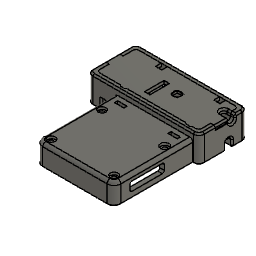
Arduino Portenta H7 and OLED Case For ML Car v32 (Autodesk Fusion 360 design; units mm, degrees)
Autodesk Fusion 360 part; units mm, degrees
note: some values were not read from the file. Chosen so that the rebuilt part matches the saved one: which face or edge a step refers to; which pieces of a blend or face edit are solid. Set by a fixed rule: which sketch regions a step uses; the direction of a hole.
(part 1 of 2)
sketch "Sketch1" plane through (0, 0, 0) normal (0, 0, 1) x (1, 0, 0)
  line L0 (1.5, 0) -> (43, 0)
  line L1 (44.5, 1.5) -> (44.5, 35.5)
  line L2 (43, 37) -> (1.5, 37)
  line L3 (0, 35.5) -> (0, 1.5)
  circle A0 centre (2, 34.875) radius 1.5
  circle A1 centre (42.5, 34.875) radius 1.5
  circle A2 centre (42.5, 2.125) radius 1.5
  circle A3 centre (2, 2.125) radius 1.5
  arc A4 (1.5, 37) -> (0, 35.5) centre (1.5, 35.5) ccw
  arc A5 (44.5, 35.5) -> (43, 37) centre (43, 35.5) ccw
  arc A6 (0, 1.5) -> (1.5, 0) centre (1.5, 1.5) ccw
  arc A7 (43, 0) -> (44.5, 1.5) centre (43, 1.5) ccw
  line L4 (1.5, -3) -> (43, -3)
  arc A8 (43, -3) -> (47.5, 1.5) centre (43, 1.5) ccw
  line L5 (47.5, 1.5) -> (47.5, 40)
  line L6 (47.5, 40) -> (-3, 40)
  line L7 (-3, 40) -> (-3, 1.5)
  arc A9 (-3, 1.5) -> (1.5, -3) centre (1.5, 1.5) ccw
  circle A10 centre (42.5, 2.125) radius 2.5
  circle A11 centre (2, 2.125) radius 2.5
  circle A12 centre (42.5, 34.875) radius 2.5
  circle A13 centre (2, 34.875) radius 2.75
  point P0 (44.5, 0)
  point P1 (0, 37)
  dimension "d1" = 44.5
  dimension "d2" = 37
  dimension "d3" = 3
  dimension "d4" = 2
  dimension "d5" = 2.125
  dimension "d6" = 2
  dimension "d7" = 2.125
  dimension "d9" = 1.5
  dimension "d16" = 1
  dimension "d17" = 1
  dimension "d19" = 1
  dimension "d372" = 5.5
  constraint horizontal L0
  constraint vertical L1
  constraint horizontal L2
  constraint vertical L3
  constraint equal A1 A3
  constraint equal A1 A2
  constraint equal A0 A2
  constraint horizontal A0.centre A1.centre
  constraint vertical A0.centre A3.centre
  constraint horizontal A2.centre A3.centre
  constraint vertical A1.centre A2.centre
  constraint coincident P1 L2
  constraint coincident P1 L3
  constraint tangent L2 A4
  constraint tangent L3 A4
  constraint tangent L1 A5
  constraint tangent L2 A5
  constraint equal A4 A5
  constraint coincident origin L0
  constraint coincident origin L3
  constraint tangent L0 A6
  constraint tangent L3 A6
  constraint equal A4 A6
  constraint coincident P0 L0
  constraint coincident P0 L1
  constraint tangent L0 A7
  constraint tangent L1 A7
  constraint equal A4 A7
  constraint parallel L0 L4
  constraint concentric A7 A8
  constraint parallel L1 L5
  constraint parallel L2 L6
  constraint parallel L3 L7
  constraint concentric A6 A9
  constraint tangent L4 A9
  constraint tangent L4 A8
  constraint tangent A8 L5
  constraint tangent L7 A9
  constraint concentric A0 A13
  measures "d1" distance of origin P0
  measures "d2" distance of origin P1
  measures "d3" diameter of A0
  measures "d4" distance of L3 A0.centre
  measures "d5" distance of L2 A0.centre
  measures "d6" distance of L1 A1.centre
  measures "d7" distance of L0 A3.centre
  measures "d9" radius of A4
  measures "d372" diameter of A13
extrude "Extrude1" add sketch "Sketch1" along normal blind 14 contours L0 L3 A6 A11 | L0 L3 A6 A11 | L0 L1 L2 L3 A10 A11 A12 A13 | L0 L1 A7 A10 | L0 L1 A7 A10 | L2 L3 A4 A13 | L2 L3 A4 A13 | L1 L2 A5 A12 | L1 L2 A5 A12 | A0 | A1 | A2 | A3 | L4 A8 L5 L6 L7 A9 makes body 1
extrude "Extrude2" cut sketch "Sketch1" along normal up to surface (10 mm away) from surface at 4 contours L0 L3 A6 A11 | L0 L1 L2 L3 A10 A11 A12 A13 | L0 L1 A7 A10 | L2 L3 A4 A13 | L1 L2 A5 A12 | A0 | A1 | A2 | A3 picked at (2.3836, 0.2209) picked at (42.1164, 0.2209) picked at (2.5264, 36.7791) picked at (42.1164, 36.7791) bodies 1
extrude "Extrude3" cut sketch "Sketch1" along normal through all contours A0 | A1 | A2 | A3 bodies 1
extrude "Extrude28" cut sketch "Sketch1" along normal blind 1.55 contours L0 L3 A6 A11 | L0 L3 A6 A11 | L0 L1 A7 A10 | L0 L1 A7 A10 | L2 L3 A4 A13 | L2 L3 A4 A13 | L1 L2 A5 A12 | L1 L2 A5 A12 bodies 1
extrude "Extrude5" add 1 faces at (30.6667, 40, 4.6667) along direction (0, 1, 0) blind 8 on bodies 1 bodies 1
sketch "Sketch3" plane through (44.5, 0, 0) normal (-1, 0, 0) x (0, -1, 0)
  line L0 (-35.5, 4) -> (-1.5, 4)
  line L1 (-1.5, 4) -> (-1.5, 14)
  line L2 (-1.5, 14) -> (-35.5, 14)
  line L3 (-35.5, 14) -> (-35.5, 4)
  line L4 (-30.75, 4) -> (-30.75, 8)
  line L5 (-29.75, 9) -> (-7.25, 9)
  line L6 (-6.25, 8) -> (-6.25, 4)
  line L7 (-6.25, 4) -> (-30.75, 4)
  arc A0 (-29.75, 9) -> (-30.75, 8) centre (-29.75, 8) ccw
  arc A1 (-6.25, 8) -> (-7.25, 9) centre (-7.25, 8) ccw
  dimension "d30" = 4.75
  dimension "d31" = 4.75
  dimension "d33" = 5
  dimension "d35" = 1
  constraint horizontal L5
  constraint vertical L6
  constraint horizontal L7
  constraint vertical L4
  constraint tangent L4 A0
  constraint tangent L5 A0
  constraint tangent L5 A1
  constraint tangent L6 A1
  constraint equal A0 A1
  constraint collinear L0 L7
  measures "d30" distance of L3 L4
  measures "d31" distance of L1 L6
  measures "d33" distance of L5 L7
  measures "d35" radius of A0
sketch "Sketch18" plane through (0, 0, 0) normal (1, 0, 0) x (0, 1, 0)
  line L0 (1.5, 4) -> (35.5, 4)
  line L1 (35.5, 4) -> (35.5, 14)
  line L2 (35.5, 14) -> (1.5, 14)
  line L3 (1.5, 14) -> (1.5, 4)
  line L4 (8.625, 4) -> (28.375, 4)
  line L5 (29.625, 5.25) -> (29.625, 8.5)
  line L6 (28.375, 9.75) -> (8.625, 9.75)
  line L7 (7.375, 8.5) -> (7.375, 5.25)
  arc A0 (8.625, 9.75) -> (7.375, 8.5) centre (8.625, 8.5) ccw
  arc A1 (29.625, 8.5) -> (28.375, 9.75) centre (28.375, 8.5) ccw
  arc A2 (28.375, 4) -> (29.625, 5.25) centre (28.375, 5.25) ccw
  arc A3 (7.375, 5.25) -> (8.625, 4) centre (8.625, 5.25) ccw
  point P0 (7.375, 4)
  point P1 (7.375, 9.75)
  point P2 (2.125, 0)
  point P3 (34.875, 0)
  dimension "d203" = 5.75
  dimension "d204" = 5.25
  dimension "d205" = 5.25
  dimension "d206" = 1.25
  constraint horizontal L4
  constraint vertical L5
  constraint horizontal L6
  constraint vertical L7
  constraint coincident L0 P0
  constraint coincident P1 L6
  constraint coincident P1 L7
  constraint tangent L6 A0
  constraint tangent L7 A0
  constraint tangent L6 A1
  constraint tangent L5 A1
  constraint equal A0 A1
  constraint tangent L4 A2
  constraint tangent L5 A2
  constraint equal A0 A2
  constraint coincident P0 L4
  constraint coincident P0 L7
  constraint tangent L4 A3
  constraint tangent L7 A3
  constraint equal A0 A3
  measures "d203" distance of P0 P1
  measures "d204" distance of L5 P3
  measures "d205" distance of L7 P2
  measures "d206" radius of A0
extrude "Extrude6" cut sketch "Sketch18" against normal through all contours L0 L4 L5 L6 L7 A0 A1 A2 A3 bodies 1
extrude "Extrude7" cut sketch "Sketch3" against normal through all contours L0 L4 L5 L6 L7 A0 A1 bodies 1
fillet "Fillet1" radius 2 5 edges at (-3, 24.75, 0) (-1.682, -1.682, 0) (22.25, -3, 0) (46.182, -1.682, 0) (47.5, 24.75, 0) on bodies 1
chamfer "Chamfer1" distance 1 angle 45 5 edges at (44.5, 30.75, 6) (44.5, 30.4571, 8.7071) (44.5, 18.5, 9) (44.5, 6.5429, 8.7071) (44.5, 6.25, 6) on bodies 1
chamfer "Chamfer2" distance 1 angle 45 5 edges at (47.5, 24.75, 14) (-3, 24.75, 14) (-1.682, -1.682, 14) (22.25, -3, 14) (46.182, -1.682, 14) on bodies 1
sketch "Sketch4" plane through (0, 0, 0) normal (0, 0, 1) x (1, 0, 0)
  line L0 (0, 0) -> (66.04, 0)
  line L1 (66.04, 0) -> (66.04, 25.4)
  line L2 (66.04, 25.4) -> (0, 25.4)
  line L3 (0, 25.4) -> (0, 0)
  circle A0 centre (2.03, 23.37) radius 1.125
  circle A1 centre (64.01, 23.37) radius 1.125
  circle A2 centre (64.01, 2.03) radius 1.125
  circle A3 centre (2.03, 2.03) radius 1.125
  circle A4 centre (64.01, 2.03) radius 1.725
  circle A5 centre (64.01, 23.37) radius 1.725
  circle A6 centre (2.03, 23.37) radius 1.725
  circle A7 centre (2.03, 2.03) radius 1.725
  line L4 (57.07, 21.63) -> (20.07, 21.63)
  line L5 (20.07, 21.63) -> (20.07, 24.03)
  line L6 (20.07, 24.03) -> (57.07, 24.03)
  line L7 (57.07, 24.03) -> (57.07, 21.63)
  line L8 (57.07, 21.63) -> (20.07, 24.03) construction
  line L9 (20.07, 21.63) -> (57.07, 24.03) construction
  line L10 (57.07, 1.37) -> (20.07, 1.37)
  line L11 (20.07, 1.37) -> (20.07, 3.77)
  line L12 (20.07, 3.77) -> (57.07, 3.77)
  line L13 (57.07, 3.77) -> (57.07, 1.37)
  line L14 (57.07, 1.37) -> (20.07, 3.77) construction
  line L15 (20.07, 1.37) -> (57.07, 3.77) construction
  line L16 (23.09, 7.91) -> (13.09, 7.91)
  line L17 (13.09, 7.91) -> (13.09, 17.91)
  line L18 (13.09, 17.91) -> (23.09, 17.91)
  line L19 (23.09, 17.91) -> (23.09, 7.91)
  line L20 (23.09, 7.91) -> (13.09, 17.91) construction
  line L21 (13.09, 7.91) -> (23.09, 17.91) construction
  line L22 (16.09, 10.91) -> (16.09, 14.91)
  line L23 (16.09, 14.91) -> (20.09, 14.91)
  line L24 (20.09, 14.91) -> (20.09, 10.91)
  line L25 (20.09, 10.91) -> (16.09, 10.91)
  line L26 (12.99, 4.695) -> (5.99, 4.695) construction
  line L27 (5.99, 4.695) -> (5.99, 0.445) construction
  line L28 (5.99, 0.445) -> (12.99, 0.445) construction
  line L29 (12.99, 0.445) -> (12.99, 4.695) construction
  line L30 (12.99, 4.695) -> (5.99, 0.445) construction
  line L31 (5.99, 4.695) -> (12.99, 0.445) construction
  line L32 (0, 8.08) -> (-1.1, 8.08)
  line L33 (-1.1, 8.08) -> (-1.1, 17.08)
  line L34 (-1.1, 17.08) -> (0, 17.08)
  line L35 (7.1, 17.08) -> (7.1, 8.08) construction
  line L36 (7.1, 8.08) -> (-1.1, 17.08) construction
  line L37 (-1.1, 8.08) -> (7.1, 17.08) construction
  line L38 (19.62, 20.705) -> (14.32, 20.705) construction
  line L39 (14.32, 20.705) -> (14.32, 24.955) construction
  line L40 (14.32, 24.955) -> (19.62, 24.955) construction
  line L41 (19.62, 24.955) -> (19.62, 20.705) construction
  line L42 (19.62, 20.705) -> (14.32, 24.955) construction
  line L43 (14.32, 20.705) -> (19.62, 24.955) construction
  line L44 (63.86, 18.41) -> (69.04, 18.41)
  line L45 (63.86, 14.41) -> (69.04, 14.41)
  arc A8 (63.86, 18.41) -> (63.86, 14.41) centre (63.86, 16.41) ccw
  arc A9 (63.86, 14.41) -> (63.86, 18.41) centre (63.86, 16.41) ccw construction
  line L46 (0, 17.08) -> (7.1, 17.08) construction
  line L47 (7.1, 8.08) -> (0, 8.08) construction
  line L48 (-3, 28.4) -> (-3, -3)
  line L49 (-3, -3) -> (69.04, -3)
  line L50 (69.04, -3) -> (69.04, 28.4)
  line L51 (69.04, 28.4) -> (-3, 28.4)
  point P0 (38.57, 22.83)
  point P1 (38.57, 2.57)
  point P2 (18.09, 12.91)
  point P3 (9.49, 2.57)
  point P4 (3, 12.58)
  point P5 (16.97, 22.83)
  dimension "d43" = 66.04
  dimension "d44" = 25.4
  dimension "d45" = 2.03
  dimension "d46" = 2.03
  dimension "d47" = 2.03
  dimension "d48" = 2.03
  dimension "d49" = 2.25
  dimension "d255" = 37
  dimension "d256" = 2.4
  dimension "d257" = 38.57
  dimension "d258" = 2.57
  dimension "d259" = 2.57
  dimension "d260" = 10
  dimension "d261" = 10
  dimension "d262" = 3
  dimension "d263" = 12.49
  dimension "d264" = 18.09
  dimension "d265" = 3.45
  dimension "d266" = 7
  dimension "d267" = 4.25
  dimension "d268" = 9.49
  dimension "d270" = 8.2
  dimension "d271" = 9
  dimension "d272" = 1.1
  dimension "d273" = 12.82
  dimension "d274" = 5.3
  dimension "d275" = 4.25
  dimension "d276" = 16.97
  dimension "d277" = 4
  dimension "d278" = 2.18
  dimension "d279" = 8.99
  dimension "d280" = 3
  constraint horizontal L0
  constraint vertical L1
  constraint horizontal L2
  constraint vertical L3
  constraint coincident L0.start L3.end
  constraint equal A0 A1
  constraint equal A1 A2
  constraint equal A2 A3
  constraint vertical A0.centre A3.centre
  constraint vertical A1.centre A2.centre
  constraint horizontal A2.centre A3.centre
  constraint horizontal A0.centre A1.centre
  constraint coincident L3.end L0
  constraint coincident L0.start L3
  constraint concentric A0 A6
  constraint concentric A3 A7
  constraint horizontal L4
  constraint perpendicular L4 L5
  constraint parallel L4 L6
  constraint parallel L5 L7
  constraint coincident L8 P0
  constraint coincident L9 P0
  constraint horizontal L10
  constraint perpendicular L10 L11
  constraint parallel L10 L12
  constraint parallel L11 L13
  constraint coincident L14 P1
  constraint coincident L15 P1
  constraint equal L4 L12
  constraint equal L5 L13
  constraint vertical P0 P1
  constraint horizontal L16
  constraint perpendicular L16 L17
  constraint parallel L16 L18
  constraint parallel L17 L19
  constraint coincident L20 P2
  constraint coincident L21 P2
  constraint equal A6 A7
  constraint equal A4 A5
  constraint equal A4 A7
  constraint coincident A1.centre A5.centre
  constraint coincident A2.centre A4.centre
  constraint horizontal L26
  constraint perpendicular L26 L27
  constraint parallel L26 L28
  constraint parallel L27 L29
  constraint coincident L30 P3
  constraint coincident L31 P3
  constraint horizontal P1 P3
  constraint horizontal L32
  constraint perpendicular L32 L33
  constraint parallel L32 L34
  constraint parallel L33 L35
  constraint coincident L36 P4
  constraint coincident L37 P4
  constraint horizontal L38
  constraint perpendicular L38 L39
  constraint parallel L38 L40
  constraint parallel L39 L41
  constraint coincident L42 P5
  constraint coincident L43 P5
  constraint horizontal P0 P5
  constraint horizontal L45
  constraint horizontal L44
  constraint tangent L45 A8
  constraint tangent L44 A8
  constraint concentric A8 A9
  constraint coincident L3 L34.end
  constraint parallel L32 L46
  constraint coincident L3 L32.start
  constraint horizontal L47
  constraint coincident L50 L44.end
  constraint coincident L50 L45.end
  measures "d43" distance of L0.start L0.end
  measures "d44" distance of L0.start L2.end
  measures "d45" distance of L3 A0.centre
  measures "d46" distance of L2 A0.centre
  measures "d47" distance of L0 A3.centre
  measures "d48" distance of L1 A1.centre
  measures "d49" diameter of A0
  measures "d255" distance of L5.end L6.end
  measures "d256" distance of L4.end L5.end
  measures "d257" distance of L3 P0
  measures "d258" distance of L2 P0
  measures "d259" distance of L0 P1
  measures "d260" distance of L17.end L18.end
  measures "d261" distance of L16.end L17.end
  measures "d263" distance of L2 P2
  measures "d264" distance of L3 P2
  measures "d265" diameter of A6
  measures "d266" distance of L27.end L28.end
  measures "d267" distance of L26.end L27.end
  measures "d268" distance of L3 P3
  measures "d270" distance of L33.end L35.start
  measures "d271" distance of L32.end L33.end
  measures "d272" distance of L3 L33
  measures "d273" distance of L2 P4
  measures "d274" distance of L39.end L40.end
  measures "d275" distance of L38.end L39.end
  measures "d276" distance of L3 P5
  measures "d277" diameter of A8
  measures "d278" distance of L1 A8.centre
  measures "d279" distance of L2 A8.centre
extrude "Extrude8" add sketch "Sketch4" along normal blind 17.8 separate body contours L0 L1 L2 L3 L44 L45 A8 | L0 L1 L2 L3 L32 L33 L34 L44 L45 L48 L49 L50 L51 | L3 L32 L33 L34 | L1 L44 L45 A8 | L1 L44 L45 L50 | A0 | A1 | A2 | A3 | A4 | A5 | A6 | A7 | L4 L5 L6 L7 | L10 L11 L12 L13 | L16 L17 L18 L19 | L22 L23 L24 L25 makes body 2
extrude "Extrude9" cut sketch "Sketch4" along normal through all from surface at 3.25 contours L0 L1 L2 L3 L44 L45 A8 | L1 L44 L45 A8 | A0 | A1 | A2 | A3 | A4 | A5 | A6 | A7 | L4 L5 L6 L7 | L10 L11 L12 L13 | L16 L17 L18 L19 | L22 L23 L24 L25 bodies 2
extrude "Extrude10" cut sketch "Sketch4" along normal through all contours A0 | A1 | A2 | A3 | L4 L5 L6 L7 | L10 L11 L12 L13 | L16 L17 L18 L19 | L22 L23 L24 L25 bodies 2
extrude "Extrude26" add sketch "Sketch4" along normal blind 0.5 draft -10 and the other way up to surface (3.25 mm away) draft 10 from surface at 3.25 separate body contours L22 L23 L24 L25 makes body 3
extrude "Extrude27" add sketch "Sketch4" along normal blind 0.5 contours L16 L17 L18 L19 bodies 2 3
extrude "Extrude11" cut sketch "Sketch4" along normal through all from surface at 3.25 contours L3 L32 L33 L34 bodies 2
sketch "Sketch6" plane through (-1.1, 0, 0) normal (1, 0, 0) x (0, 1, 0)
  line L0 (17.08, 3.25) -> (17.08, 6.5)
  line L1 (17.08, 6.5) -> (8.08, 6.5)
  line L2 (8.08, 6.5) -> (8.08, 3.25)
  line L3 (17.08, 3.25) -> (8.08, 3.25)
  line L4 (17.08, 17.8) -> (8.08, 17.8)
  line L5 (8.08, 17.8) -> (8.08, 3.25)
  line L6 (8.08, 3.25) -> (17.08, 3.25)
  line L7 (17.08, 3.25) -> (17.08, 17.8)
  dimension "d75" = 9
  dimension "d76" = 3.25
  constraint vertical L0
  constraint horizontal L1
  constraint vertical L2
  constraint horizontal L3
  constraint collinear L2 L5
  constraint collinear L3 L6
  measures "d75" distance of L2.end L0.start
  measures "d76" distance of L2.end L1.end
extrude "Extrude12" cut sketch "Sketch6" against normal through all contours L0 L1 L2 L3 L5 L6 L7 bodies 2
fillet "Fillet2" radius 1 4 edges at (-2.05, 8.08, 6.5) (-1.5, 8.08, 3.25) (-2.05, 17.08, 6.5) (-1.5, 17.08, 3.25) on bodies 2
chamfer "Chamfer4" distance 1 angle 45 8 edges at (38.57, 3.77, 3.25) (20.07, 2.57, 3.25) (38.57, 1.37, 3.25) (57.07, 2.57, 3.25) (38.57, 21.63, 3.25) (57.07, 22.83, 3.25) (38.57, 24.03, 3.25) (20.07, 22.83, 3.25) on bodies 2
sketch "Sketch7" plane through (0, 25.4, 0) normal (0, -1, 0) x (1, 0, 0)
  line L0 (66.04, 17.8) -> (0, 17.8)
  line L1 (0, 3.25) -> (66.04, 3.25)
  line L2 (0, 17.8) -> (0, 3.25)
  line L3 (66.04, 3.25) -> (66.04, 17.8)
  line L4 (66.04, 17.8) -> (0, 17.8)
  line L5 (0, 17.8) -> (0, 3.25)
  line L6 (0, 3.25) -> (66.04, 3.25)
  line L7 (66.04, 3.25) -> (66.04, 17.8)
  line L8 (1.7344, 6.45) -> (16.7344, 6.45) construction
  line L9 (14.32, 0) -> (19.62, 0) construction
  line L10 (19.62, 6.45) -> (14.32, 6.45)
  line L11 (14.32, 6.45) -> (14.32, 3.25)
  line L12 (14.32, 3.25) -> (19.62, 3.25)
  line L13 (19.62, 3.25) -> (19.62, 6.45)
  dimension "d285" = 15
  dimension "d286" = 3.2
  constraint horizontal L8
  constraint horizontal L10
  constraint vertical L11
  constraint horizontal L12
  constraint vertical L13
  constraint vertical L9.end L12.end
  constraint vertical L9.start L11.end
  constraint collinear L8 L10
  constraint collinear L1 L12
  measures "d285" distance of L8.start L8.end
  measures "d286" distance of L1 L8
extrude "Extrude13" cut sketch "Sketch7" against normal through all contours L1 L6 L10 L11 L12 L13 bodies 2
sketch "Sketch8" plane through (0, 0, 0) normal (0, 1, 0) x (-1, 0, 0)
  line L0 (0, 17.8) -> (-66.04, 17.8)
  line L1 (-66.04, 3.25) -> (0, 3.25)
  line L2 (-66.04, 17.8) -> (-66.04, 3.25)
  line L3 (0, 3.25) -> (0, 17.8)
  line L4 (0, 17.8) -> (-66.04, 17.8)
  line L5 (-66.04, 17.8) -> (-66.04, 3.25)
  line L6 (-66.04, 3.25) -> (0, 3.25)
  line L7 (0, 3.25) -> (0, 17.8)
  line L8 (-5.99, 0) -> (-12.99, 0)
  line L9 (-4.6088, 6.45) -> (-19.6088, 6.45) construction
  line L10 (-5.99, 6.45) -> (-12.99, 6.45)
  line L11 (-12.99, 6.45) -> (-12.99, 3.25)
  line L12 (-12.99, 3.25) -> (-5.99, 3.25)
  line L13 (-5.99, 3.25) -> (-5.99, 6.45)
  dimension "d288" = 15
  dimension "d289" = 3.2
  constraint horizontal L9
  constraint horizontal L10
  constraint vertical L11
  constraint horizontal L12
  constraint vertical L13
  constraint coincident L6 L11.end
  constraint coincident L9 L10.start
  constraint vertical L8.start L12.end
  constraint vertical L8.end L11.end
  measures "d288" distance of L9.start L9.end
  measures "d289" distance of L1 L9
extrude "Extrude14" cut sketch "Sketch8" against normal through all contours L1 L6 L10 L11 L12 L13 bodies 2
chamfer "Chamfer5" distance 1 angle 45 8 edges at (9.49, -3, 3.25) (12.99, -3, 4.85) (9.49, -3, 6.45) (5.99, -3, 4.85) (14.32, 28.4, 4.85) (16.97, 28.4, 3.25) (19.62, 28.4, 4.85) (16.97, 28.4, 6.45) on bodies 2
extrude "Extrude15" cut sketch "Sketch4" along normal blind 1.5 contours A4 | A5 | A6 | A7 bodies 2
sketch "Sketch9" plane through (-3, 0, 0) normal (-1, 0, 0) x (0, -1, 0)
  line L0 (-16.08, 8.5) -> (-9.08, 8.5)
  line L1 (-6.08, 5.5) -> (-6.08, 4.25)
  line L2 (-9.08, 1.25) -> (-16.08, 1.25)
  line L3 (-19.08, 4.25) -> (-19.08, 5.5)
  arc A0 (-16.08, 8.5) -> (-19.08, 5.5) centre (-16.08, 5.5) ccw
  arc A1 (-6.08, 5.5) -> (-9.08, 8.5) centre (-9.08, 5.5) ccw
  arc A2 (-9.08, 1.25) -> (-6.08, 4.25) centre (-9.08, 4.25) ccw
  arc A3 (-19.08, 4.25) -> (-16.08, 1.25) centre (-16.08, 4.25) ccw
  line L4 (-16.08, 6.5) -> (-9.08, 6.5)
  arc A4 (-8.08, 5.5) -> (-9.08, 6.5) centre (-9.08, 5.5) ccw
  line L5 (-8.08, 5.5) -> (-8.08, 4.25)
  arc A5 (-9.08, 3.25) -> (-8.08, 4.25) centre (-9.08, 4.25) ccw
  line L6 (-9.08, 3.25) -> (-16.08, 3.25)
  arc A6 (-17.08, 4.25) -> (-16.08, 3.25) centre (-16.08, 4.25) ccw
  line L7 (-17.08, 4.25) -> (-17.08, 5.5)
  arc A7 (-16.08, 6.5) -> (-17.08, 5.5) centre (-16.08, 5.5) ccw
  line L8 (-9.08, 6.5) -> (-16.08, 6.5)
  arc A8 (-16.08, 6.5) -> (-17.08, 5.5) centre (-16.08, 5.5) ccw
  line L9 (-17.08, 5.5) -> (-17.08, 17.8)
  line L10 (-17.08, 17.8) -> (-8.08, 17.8)
  line L11 (-8.08, 17.8) -> (-8.08, 5.5)
  arc A9 (-8.08, 5.5) -> (-9.08, 6.5) centre (-9.08, 5.5) ccw
  point P0 (-12.58, 17.8)
  point P1 (-12.58, 6.5)
  point P2 (-12.58, 8.5)
  point P3 (-8.08, 4.875)
  point P4 (-6.08, 4.875)
  dimension "d101" = 3
  constraint horizontal L0
  constraint vertical L1
  constraint horizontal L2
  constraint vertical L3
  constraint tangent L0 A0
  constraint tangent L3 A0
  constraint tangent L0 A1
  constraint tangent L1 A1
  constraint equal A0 A1
  constraint tangent L1 A2
  constraint tangent L2 A2
  constraint equal A0 A2
  constraint tangent L2 A3
  constraint tangent L3 A3
  constraint equal A0 A3
  constraint midpoint L10 P0
  constraint midpoint L4 P1
  constraint midpoint L0 P2
  constraint vertical P1 P2
  constraint midpoint L5 P3
  constraint midpoint L1 P4
  constraint horizontal P3 P4
  measures "d101" radius of A0
extrude "Extrude16" cut sketch "Sketch9" against normal blind 0.75 contours L0 A0 A1 L4 A4 A7 L8 A8 L9 L11 A9 | L1 L2 L3 A0 A1 A2 A3 L5 A5 L6 A6 L7 L9 L11 bodies 2
chamfer "Chamfer7" distance 0.5 angle 45 8 edges at (-2.25, 12.58, 3.25) (-2.25, 8.3729, 3.5429) (-2.25, 8.08, 4.875) (-2.25, 8.3729, 6.2071) (-2.25, 12.58, 6.5) (-2.25, 16.7871, 6.2071) (-2.25, 17.08, 4.875) (-2.25, 16.7871, 3.5429) on bodies 2
sketch "Sketch11" plane through (0, 0, 17.8) normal (0, 0, 1) x (-1, 0, 0)
  line L0 (-61.82, 0) -> (-61.07, 0.75)
  line L1 (-61.07, 0.75) -> (-58.57, 0.75)
  line L2 (-58.57, 0.75) -> (-57.82, 0)
  line L3 (0, 0) -> (-66.04, 0)
  line L4 (1.1, -17.08) -> (0, -17.08)
  line L5 (0, -17.08) -> (0, -25.4)
  line L6 (0, -25.4) -> (-66.04, -25.4)
  line L7 (-66.04, -25.4) -> (-66.04, 0)
  line L8 (-66.04, 0) -> (0, 0)
  line L9 (0, 0) -> (0, -8.08)
  line L10 (0, -8.08) -> (1.1, -8.08)
  line L11 (1.1, -8.08) -> (1.1, -17.08)
  line L12 (-69.04, -28.4) -> (3, -28.4)
  line L13 (3, -28.4) -> (3, 3)
  line L14 (3, 3) -> (-69.04, 3)
  line L15 (-69.04, 3) -> (-69.04, -28.4)
  line L16 (-20.07, -1.37) -> (-20.07, -3.77)
  line L17 (-57.07, -3.77) -> (-57.07, -1.37)
  line L18 (-19.32, 0) -> (-18.57, 0.75)
  line L19 (-18.57, 0.75) -> (-16.07, 0.75)
  line L20 (-16.07, 0.75) -> (-15.32, 0)
  point P0 (-12.99, 0)
  dimension "d105" = 135
  dimension "d107" = 2.5
  dimension "d108" = 0.75
  dimension "d293" = 0.75
  dimension "d294" = 0.75
  dimension "d295" = 2.5
  constraint perpendicular L0 L2
  constraint horizontal L1
  constraint coincident L2.end L8
  constraint coincident L0.start L8
  constraint coincident L3 L18.start
  constraint coincident L3 L20.end
  constraint collinear L1 L19
  constraint parallel L2 L20
  constraint parallel L0 L18
  measures "d105" angle of L1 L2
  measures "d107" distance of L0.end L1.end
  measures "d108" distance of L1 L3
  measures "d293" distance of L2.end L17
  measures "d294" horizontal distance of L16.end L18.start
  measures "d295" distance of L18.end L19.end
extrude "Extrude17" cut sketch "Sketch11" against normal up to surface (14.55 mm away) contours L0 L1 L2 L3 L8 | L3 L8 L18 L19 L20 bodies 2
sketch "Sketch14" plane through (0, 0, 3.25) normal (0, 0, 1) x (-1, 0, 0)
  circle A0 centre (-1.5, -19.3644) radius 1.5
  circle A1 centre (-2.25, -6.1356) radius 1.5
  line L0 (1.75, -12.75) -> (-32.3092, -12.75) construction
  line L1 (-1.5, -19.3644) -> (-2.25, -6.1356) construction
  line L2 (1.75, -9.08) -> (0, -9.08)
  line L3 (0, -9.08) -> (0, 0)
  line L4 (0, 0) -> (-5.99, 0)
  line L5 (-5.99, 0) -> (-5.99, 2)
  line L6 (-5.99, 2) -> (-12.99, 2)
  line L7 (-12.99, 2) -> (-12.99, 0)
  line L8 (-12.99, 0) -> (-15.32, 0)
  line L9 (-15.32, 0) -> (-16.07, 0.75)
  line L10 (-16.07, 0.75) -> (-18.57, 0.75)
  line L11 (-18.57, 0.75) -> (-19.32, 0)
  line L12 (-19.32, 0) -> (-57.82, 0)
  line L13 (-57.82, 0) -> (-58.57, 0.75)
  line L14 (-58.57, 0.75) -> (-61.07, 0.75)
  line L15 (-61.07, 0.75) -> (-61.82, 0)
  line L16 (-61.82, 0) -> (-66.04, 0)
  line L17 (-66.04, 0) -> (-66.04, -25.4)
  line L18 (-66.04, -25.4) -> (-19.62, -25.4)
  line L19 (-19.62, -25.4) -> (-19.62, -27.4)
  line L20 (-19.62, -27.4) -> (-14.32, -27.4)
  line L21 (-14.32, -27.4) -> (-14.32, -25.4)
  line L22 (-14.32, -25.4) -> (0, -25.4)
  line L23 (0, -25.4) -> (0, -16.08)
  line L24 (-58.07, -25.03) -> (-58.07, -20.63)
  line L25 (-58.07, -20.63) -> (-19.07, -20.63)
  line L26 (-19.07, -20.63) -> (-19.07, -25.03)
  line L27 (-19.07, -25.03) -> (-58.07, -25.03)
  circle A2 centre (-64.01, -2.03) radius 1.125
  circle A3 centre (-2.03, -23.37) radius 1.125
  circle A4 centre (-64.01, -23.37) radius 1.125
  circle A5 centre (-2.03, -2.03) radius 1.125
  line L28 (-13.09, -7.91) -> (-13.09, -17.91)
  line L29 (-13.09, -17.91) -> (-23.09, -17.91)
  line L30 (-23.09, -17.91) -> (-23.09, -7.91)
  line L31 (-23.09, -7.91) -> (-13.09, -7.91)
  line L32 (-19.07, -0.37) -> (-19.07, -4.77)
  line L33 (-19.07, -4.77) -> (-58.07, -4.77)
  line L34 (-58.07, -4.77) -> (-58.07, -0.37)
  line L35 (-58.07, -0.37) -> (-19.07, -0.37)
  line L36 (0, -16.08) -> (1.75, -16.08)
  line L37 (1.75, -16.08) -> (1.75, -9.08)
  point P0 (-1.875, -12.75)
  point P1 (-1.875, -12.75)
  dimension "d144" = 3
  dimension "d145" = 13.25
  constraint equal A0 A1
  constraint coincident A0.centre L1.start
  constraint coincident A1.centre L1.end
  constraint coincident L0 P1
  constraint midpoint L1 P1
  constraint coincident P1 P0
  measures "d144" diameter of A0
  measures "d145" distance of A0.centre A1.centre
sketch "Sketch15" plane through (0, 0, 0) normal (0, 0, -1) x (1, 0, 0)
  circle A0 centre (2.25, -6.1356) radius 0.6
  circle A1 centre (1.5, -19.3644) radius 0.6
  circle A2 centre (2.25, -6.1356) radius 1.5
  circle A3 centre (1.5, -19.3644) radius 1.5
  circle A4 centre (2.03, -23.37) radius 1.725
  circle A5 centre (64.01, -23.37) radius 1.725
  circle A6 centre (2.03, -2.03) radius 1.725
  circle A7 centre (64.01, -2.03) radius 1.725
  line L0 (20.07, -24.03) -> (20.07, -21.63)
  line L1 (20.07, -21.63) -> (57.07, -21.63)
  line L2 (57.07, -21.63) -> (57.07, -24.03)
  line L3 (57.07, -24.03) -> (20.07, -24.03)
  line L4 (20.07, -3.77) -> (20.07, -1.37)
  line L5 (20.07, -1.37) -> (57.07, -1.37)
  line L6 (57.07, -1.37) -> (57.07, -3.77)
  line L7 (57.07, -3.77) -> (20.07, -3.77)
  line L8 (-3, -28.4) -> (69.04, -28.4)
  line L9 (69.04, -28.4) -> (69.04, 3)
  line L10 (69.04, 3) -> (-3, 3)
  line L11 (-3, 3) -> (-3, -28.4)
  dimension "d151" = 1.2
  constraint equal A0 A1
  constraint concentric A0 A2
  constraint concentric A1 A3
  measures "d151" diameter of A0
fillet "Fillet5" radius 2 4 edges at (0, 25.4, 10.525) (0, 0, 10.525) (66.04, 0, 10.525) (66.04, 25.4, 10.525) on bodies 2
fillet "Fillet5" radius 3.5 4 edges at (69.04, -3, 8.9) (69.04, 28.4, 8.9) (-3, -3, 8.9) (-3, 28.4, 8.9) on bodies 2
loft "Loft1" cut profiles "Sketch14", "Sketch15" section 1 contours A0 section 2 contours A1 bodies 2
loft "Loft2" cut profiles "Sketch14", "Sketch15" section 1 contours A1 section 2 contours A0 bodies 2
sketch "Sketch10" plane through (0, 0, 17.8) normal (0, 0, 1) x (-1, 0, 0)
  line L0 (-65.54, -28.4) -> (-0.5, -28.4)
  line L1 (3, -24.9) -> (3, -0.5)
  line L2 (-0.5, 3) -> (-65.54, 3)
  line L3 (-69.04, -0.5) -> (-69.04, -24.9)
  line L4 (-61.82, 0) -> (-61.07, 0.75)
  line L5 (-61.07, 0.75) -> (-58.57, 0.75)
  line L6 (-58.57, 0.75) -> (-57.82, 0)
  line L7 (-57.82, 0) -> (-19.32, 0)
  line L8 (-19.32, 0) -> (-18.57, 0.75)
  line L9 (-18.57, 0.75) -> (-16.07, 0.75)
  line L10 (-16.07, 0.75) -> (-15.32, 0)
  line L11 (-15.32, 0) -> (-2, 0)
  arc A0 (0, -2) -> (-2, 0) centre (-2, -2) ccw
  line L12 (0, -2) -> (0, -8.08)
  line L13 (0, -8.08) -> (1.1, -8.08)
  line L14 (1.1, -8.08) -> (1.1, -17.08)
  line L15 (1.1, -17.08) -> (0, -17.08)
  line L16 (0, -17.08) -> (0, -23.4)
  arc A1 (-2, -25.4) -> (0, -23.4) centre (-2, -23.4) ccw
  line L17 (-2, -25.4) -> (-64.04, -25.4)
  arc A2 (-66.04, -23.4) -> (-64.04, -25.4) centre (-64.04, -23.4) ccw
  line L18 (-66.04, -23.4) -> (-66.04, -2)
  arc A3 (-64.04, 0) -> (-66.04, -2) centre (-64.04, -2) ccw
  line L19 (-64.04, 0) -> (-61.82, 0)
  line L20 (-20.31, -21.75) -> (-16.31, -21.75)
  line L21 (-16.31, -21.75) -> (-16.31, -25.4)
  line L22 (-16.31, -24.75) -> (-20.31, -24.75) construction
  line L23 (-20.31, -25.4) -> (-20.31, -21.75)
  line L24 (-20.31, -21.75) -> (-16.31, -24.75) construction
  line L25 (-16.31, -21.75) -> (-20.31, -24.75) construction
  line L26 (-57.98, -21.75) -> (-53.98, -21.75)
  line L27 (-53.98, -21.75) -> (-53.98, -25.4)
  line L28 (-53.98, -24.75) -> (-57.98, -24.75) construction
  line L29 (-57.98, -25.4) -> (-57.98, -21.75)
  line L30 (-57.98, -21.75) -> (-53.98, -24.75) construction
  line L31 (-53.98, -21.75) -> (-57.98, -24.75) construction
  circle A4 centre (-38.65, -13.34) radius 2.5
  line L32 (-22.53, 1.1447) -> (-33.6, 1.1447) construction
  line L33 (-33.58, 2.1447) -> (-22.55, 2.1447) construction
  line L34 (-22.55, 2.1447) -> (-22.55, 0.1447) construction
  line L35 (-22.55, 0.1447) -> (-33.58, 0.1447) construction
  line L36 (-33.58, 0.1447) -> (-33.58, 2.1447) construction
  line L37 (-33.58, 2.1447) -> (-22.55, 0.1447) construction
  line L38 (-22.55, 2.1447) -> (-33.58, 0.1447) construction
  line L39 (-63.71, -20.52) -> (-69.04, -20.52)
  line L40 (-63.71, -16.52) -> (-69.04, -16.52)
  arc A5 (-63.71, -20.52) -> (-63.71, -16.52) centre (-63.71, -18.52) ccw
  arc A6 (-63.71, -16.52) -> (-63.71, -20.52) centre (-63.71, -18.52) ccw construction
  line L41 (-26.95, -16.59) -> (-30.4, -16.59)
  line L42 (-30.4, -16.59) -> (-30.4, -3.97)
  line L43 (-30.4, -3.97) -> (-26.95, -3.97)
  line L44 (-26.95, -3.97) -> (-26.95, -16.59)
  circle A7 centre (-38.65, -13.34) radius 1.875 construction
  circle A8 centre (-64.01, -2.03) radius 1.125
  circle A9 centre (-64.01, -2.03) radius 1.125
  circle A10 centre (-64.01, -23.37) radius 1.125
  circle A11 centre (-2.03, -23.37) radius 1.125
  circle A12 centre (-2.03, -2.03) radius 1.125
  circle A13 centre (-2.03, -2.03) radius 0.875
  circle A14 centre (-64.01, -2.03) radius 0.875
  circle A15 centre (-64.01, -23.37) radius 0.875
  circle A16 centre (-2.03, -23.37) radius 0.875
  line L45 (1.1, -17.08) -> (3, -17.08)
  line L46 (1.1, -8.08) -> (3, -8.08)
  arc A17 (-0.5, -28.4) -> (3, -24.9) centre (-0.5, -24.9) ccw
  arc A18 (3, -0.5) -> (-0.5, 3) centre (-0.5, -0.5) ccw
  arc A19 (-65.54, 3) -> (-69.04, -0.5) centre (-65.54, -0.5) ccw
  arc A20 (-69.04, -24.9) -> (-65.54, -28.4) centre (-65.54, -24.9) ccw
  line L47 (-36.15, -15.84) -> (-41.15, -15.84)
  line L48 (-41.15, -15.84) -> (-41.15, -10.84)
  line L49 (-41.15, -10.84) -> (-36.15, -10.84)
  line L50 (-36.15, -10.84) -> (-36.15, -15.84)
  point P0 (-18.31, -23.25)
  point P1 (-55.98, -23.25)
  point P2 (-28.065, 1.1447)
  point P3 (-28.065, 1.1447)
  dimension "d306" = 4
  dimension "d307" = 3
  dimension "d308" = 18.31
  dimension "d309" = 2.15
  dimension "d310" = 10.06
  dimension "d311" = 5
  dimension "d312" = 12.06
  dimension "d313" = 38.65
  dimension "d315" = 32.44
  dimension "d316" = 22.53
  dimension "d317" = 11.03
  dimension "d318" = 2
  dimension "d319" = 4
  dimension "d320" = 2.33
  dimension "d321" = 6.88
  dimension "d322" = 3.45
  dimension "d323" = 12.62
  dimension "d324" = 8.25
  dimension "d325" = 3.25
  dimension "d326" = 3.75
  dimension "d327" = 2.25
  dimension "d329" = 1.75
  constraint horizontal L20
  constraint perpendicular L20 L21
  constraint parallel L20 L22
  constraint parallel L21 L23
  constraint coincident L24 P0
  constraint coincident L25 P0
  constraint horizontal L26
  constraint perpendicular L26 L27
  constraint parallel L26 L28
  constraint parallel L27 L29
  constraint coincident L30 P1
  constraint coincident L31 P1
  constraint horizontal P0 P1
  constraint equal L22 L28
  constraint horizontal L32
  constraint midpoint L32 P3
  constraint horizontal L33
  constraint perpendicular L33 L34
  constraint parallel L33 L35
  constraint parallel L34 L36
  constraint coincident L37 P3
  constraint coincident L38 P3
  constraint coincident P3 P2
  constraint tangent L39 A5
  constraint tangent L40 A5
  constraint horizontal L39
  constraint horizontal L40
  constraint coincident L3 L39.end
  constraint coincident L3 L40.end
  constraint concentric A5 A6
  constraint horizontal L41
  constraint vertical L42
  constraint horizontal L43
  constraint vertical L44
  constraint concentric A4 A7
  constraint concentric A12 A13
  constraint concentric A9 A14
  constraint concentric A10 A15
  constraint concentric A11 A16
  constraint equal A15 A16
  constraint equal A14 A15
  constraint equal A13 A14
  constraint coincident L14.end L15.start
  constraint coincident L1 L45.end
  constraint coincident L13.end L14.start
  constraint coincident L1 L46.end
  constraint horizontal L45
  constraint horizontal L46
  constraint coincident L17 L29.start
  constraint coincident L28.end L29
  constraint coincident L17 L27.end
  constraint coincident L28.start L27
  constraint coincident L17 L23.start
  constraint coincident L22.end L23
  constraint coincident L17 L21.end
  constraint coincident L22.start L21
  constraint horizontal L20.start L26.end
  constraint horizontal L47
  constraint vertical L48
  constraint horizontal L49
  constraint vertical L50
  constraint tangent A4 L47
  constraint tangent A4 L50
  constraint tangent A4 L48
  constraint tangent A4 L49
  measures "d306" distance of L22.start L22.end
  measures "d307" distance of L20.end L22.start
  measures "d308" distance of L16 P0
  measures "d309" distance of L17 P0
  measures "d310" distance of L18 P1
  measures "d311" diameter of A4
  measures "d312" distance of L17 A4.centre
  measures "d313" distance of L16 A4.centre
  measures "d315" distance of L18 L32.end
  measures "d316" distance of L12 L32.start
  measures "d317" distance of L34.end L35.end
  measures "d318" distance of L33.end L34.end
  measures "d319" diameter of A5
  measures "d320" distance of L18 A5.centre
  measures "d321" distance of L17 A5.centre
  measures "d322" distance of L41.start L41.end
  measures "d323" distance of L41.start L43.end
  measures "d324" distance of A4.centre L42
  measures "d325" distance of A4.centre L41
  measures "d326" diameter of A7
  measures "d327" diameter of A8
  measures "d329" diameter of A13
extrude "Extrude18" add sketch "Sketch10" against normal blind 2.5 separate body contours L4 L5 L6 L7 L8 L9 L10 L11 A0 L12 L13 L14 L15 L16 A1 L17 A2 L18 A3 L19 L20 L21 L23 L26 L27 L29 L39 L40 A5 | A4 L47 L50 | A4 L49 L50 | A4 L48 L49 | A4 L47 L48 | A8 A9 | A10 | A11 | A12 | A13 | A14 | A15 | A16 makes body 4
extrude "Extrude20" cut sketch "Sketch10" against normal through all from surface at -1 contours A13 | A14 | A15 | A16 bodies 4
sketch "Sketch13" plane through (66.04, 0, 0) normal (1, 0, 0) x (0, 1, 0)
  line L0 (23.5, 15.3) -> (23.5, 17.8)
  line L1 (23.5, 17.8) -> (2, 17.8)
  line L2 (2, 17.8) -> (2, 15.3)
  line L3 (7.75, 17.8) -> (17.75, 17.8)
  line L4 (17.75, 17.8) -> (17.75, 15.3)
  line L5 (17.75, 15.3) -> (7.75, 15.3)
  line L6 (7.75, 15.3) -> (7.75, 17.8)
  line L7 (2, 16.55) -> (23.5, 16.55) construction
  line L8 (2, 15.3) -> (23.5, 15.3)
  line L9 (25.4, 17.8) -> (0, 17.8)
  line L10 (0, 17.8) -> (0, 15.3)
  line L11 (0, 15.3) -> (25.4, 15.3)
  line L12 (25.4, 15.3) -> (25.4, 17.8)
  line L13 (16.52, 17.8) -> (2, 17.8)
  line L14 (2, 17.8) -> (2, 15.3)
  line L15 (2, 15.3) -> (16.52, 15.3)
  line L16 (16.52, 15.3) -> (16.52, 17.8)
  point P0 (12.75, 17.8)
  point P1 (12.75, 16.55)
  dimension "d139" = 10
  constraint horizontal L3
  constraint vertical L4
  constraint horizontal L5
  constraint vertical L6
  constraint coincident L1 L3.start
  constraint midpoint L2 L7.start
  constraint midpoint L0 L7.end
  constraint midpoint L3 P0
  constraint midpoint L7 P1
  constraint vertical P0 P1
  constraint horizontal L0.start L4.end
  measures "d139" distance of L3.start L3.end
extrude "Extrude21" add sketch "Sketch13" along normal up to surface (3 mm away) contours L1 L3 L5 L6 L8 L9 L11 L13 L15 L16 bodies 4
extrude "Extrude22" cut sketch "Sketch13" along normal through all contours L1 L3 L5 L6 L8 L9 L11 L13 L15 L16 bodies 2
extrude "Extrude30" add 1 faces at (-1.1, 11.08, 16.9667) along direction (-1, 0, 0) up to surface (1.9 mm away) on bodies 4 bodies 4
extrude "Extrude31" cut 1 faces at (-3, 11.08, 16.9667) along direction (1, 0, 0) up to surface (3 mm away) on bodies 4 bodies 2
extrude "Extrude36" cut sketch "Sketch10" against normal through all from surface at -0.5 contours A4 | A4 L47 L50 | A4 L49 L50 | A4 L48 L49 | A4 L47 L48 bodies 4
chamfer "Chamfer9" distance 0.5 angle 45 39 edges at (38.57, 0, 15.3) (17.32, -0.75, 15.3) (15.695, -0.375, 15.3) (18.945, -0.375, 15.3) (58.195, -0.375, 15.3) (59.82, -0.75, 15.3) (61.445, -0.375, 15.3) (67.54, 7.75, 15.3) (-1.5, 17.08, 15.3) (-1.5, 8.08, 15.3) (-3, 12.58, 15.3) (69.04, 12.135, 15.3) (30.4, 10.28, 15.3) (28.675, 3.97, 15.3) (26.95, 10.28, 15.3) (28.675, 16.59, 15.3) (8.66, 0, 15.3) (0.5858, 0.5858, 15.3) (0, 5.04, 15.3) (0, 20.24, 15.3) (0.5858, 24.8142, 15.3) (9.155, 25.4, 15.3) (61.01, 25.4, 15.3) (65.4542, 24.8142, 15.3) (66.04, 21.96, 15.3) (37.145, 25.4, 15.3) (65.4542, 0.5858, 15.3) (66.04, 4.875, 15.3) (62.93, 0, 15.3) (36.15, 13.34, 15.3) (38.65, 10.84, 15.3) (38.65, 15.84, 15.3) (41.15, 13.34, 15.3) (53.98, 23.575, 15.3) (55.98, 21.75, 15.3) (57.98, 23.575, 15.3) (16.31, 23.575, 15.3) (18.31, 21.75, 15.3) (20.31, 23.575, 15.3) on bodies 4
chamfer "Chamfer9" distance 0.2 angle 45 4 faces at (36.6412, 11.3312, 17.3) (36.6412, 15.3488, 17.3) (40.6588, 15.3488, 17.3) (40.6588, 11.3312, 17.3) on bodies 4
sketch "Sketch17" plane through (0, -3, 0) normal (0, -1, 0) x (1, 0, 0)
  line L0 (13.99, 6.4799) -> (65.54, 6.4799) construction
  line L1 (65.54, 6.4799) -> (65.54, 0) construction
  line L2 (65.54, 0) -> (13.99, 0) construction
  line L3 (13.99, 0) -> (13.99, 6.4799) construction
  line L4 (39.765, 6.4799) -> (39.765, 0) construction
  line L5 (16.6, 14) -> (63.1, 14)
  line L6 (65.1, 12) -> (65.1, 1)
  line L7 (64.1, 0) -> (15.6, 0)
  line L8 (14.6, 1) -> (14.6, 12)
  line L9 (39.765, 14) -> (39.765, 0) construction
  arc A0 (65.1, 12) -> (63.1, 14) centre (63.1, 12) ccw
  arc A1 (16.6, 14) -> (14.6, 12) centre (16.6, 12) ccw
  line L10 (65.1, 1) -> (64.1, 0)
  line L11 (15.6, 0) -> (14.6, 1)
  line L12 (0.5, 0) -> (65.54, 0)
  line L13 (65.54, 17.8) -> (0.5, 17.8)
  line L14 (13.99, 2.25) -> (4.99, 2.25)
  line L15 (4.99, 2.25) -> (4.99, 7.45)
  line L16 (4.99, 7.45) -> (13.99, 7.45)
  line L17 (13.99, 7.45) -> (13.99, 2.25)
  line L18 (0.5, 17.8) -> (0.5, 0)
  line L19 (65.54, 0) -> (65.54, 17.8)
  point P0 (14.6, 10)
  point P1 (65.1, 10)
  point P2 (14.6, 14)
  point P3 (65.1, 14)
  point P4 (65.1, 0)
  point P5 (14.6, 0)
  dimension "d196" = 50.5
  dimension "d207" = 50.5
  dimension "d208" = 14
  dimension "d209" = 2
  dimension "d210" = 1
  dimension "d211" = 1
  dimension "d212" = 1
  dimension "d213" = 1
  constraint horizontal L0
  constraint vertical L1
  constraint horizontal L2
  constraint vertical L3
  constraint midpoint L0 L4.start
  constraint midpoint L2 L4.end
  constraint horizontal L5
  constraint vertical L6
  constraint horizontal L7
  constraint vertical L8
  constraint collinear L4 L9
  constraint collinear L2 L7
  constraint coincident L5 L9.start
  constraint coincident P3 L5
  constraint coincident P3 L6
  constraint tangent L5 A0
  constraint tangent L6 A0
  constraint coincident P2 L5
  constraint coincident P2 L8
  constraint tangent L5 A1
  constraint tangent L8 A1
  constraint equal A0 A1
  constraint coincident L7 L4.end
  constraint coincident P4 L6
  constraint coincident P4 L7
  constraint coincident P5 L7
  constraint coincident P5 L8
  constraint collinear L3 L17
  constraint collinear L1 L19
  constraint collinear L7 L12
  measures "d196" distance of P0 P1
  measures "d207" distance of P2 P3
  measures "d208" distance of P2 P5
  measures "d209" radius of A0
  measures "d210" distance of P4 L6.end
  measures "d211" distance of P4 L7.start
  measures "d212" distance of P5 L7.end
  measures "d213" distance of P5 L8.start
move_body "Move3" bodies 1 to x (-1, 0, 0) y (0, 1, 0) z (0, 0, -1) at (44.5, 0, 10)
move_body "Move2" bodies 1 to x (1, 0, 0) y (0, 1, 0) z (0, 0, 1) at (17.6, -51, 4)
combine "Combine1" operation add target body 1 tool bodies 2
chamfer "Chamfer10" distance 1 angle 45 9 edges at (8.05, -3, 0) (64.82, -3, 0) (68.0149, -1.9749, 0) (69.04, 12.7, 0) (68.0149, 27.3749, 0) (33.02, 28.4, 0) (-1.9749, 27.3749, 0) (-3, 12.7, 0) (-1.9749, -1.9749, 0) on bodies 1
split "Split1" by plane through (-3, -3, 0) normal (0, -1, 0) bodies 1 makes body 5 at (33.6498, -27.6652, 14)
sketch "Sketch19" plane through (0, -3, 0) normal (0, -1, 0) x (-1, 0, 0)
  line L0 (-57.1, -4) -> (-22.6, -4) construction
  line L1 (-39.85, 0) -> (-39.85, -14) construction
  line L2 (-64.1, 0) -> (-65.1, -1)
  line L3 (-65.1, -1) -> (-65.54, -1)
  line L4 (-65.54, -1) -> (-65.54, -17.8)
  line L5 (-13.99, -2.25) -> (-4.99, -2.25)
  line L6 (-4.99, -2.25) -> (-4.99, -7.45)
  line L7 (-4.99, -7.45) -> (-13.99, -7.45)
  line L8 (-13.99, -7.45) -> (-13.99, -2.25)
  line L9 (-14.6, -1) -> (-15.6, 0)
  line L10 (-15.6, 0) -> (-64.1, 0)
  line L11 (-64.1, 0) -> (-65.1, -1)
  line L12 (-65.1, -1) -> (-65.54, -1)
  line L13 (-65.54, -1) -> (-65.54, -17.8)
  line L14 (-65.54, -17.8) -> (-0.5, -17.8)
  line L15 (-0.5, -17.8) -> (-0.5, -1)
  line L16 (-0.5, -1) -> (-14.6, -1)
  line L17 (-15.6, 0) -> (-14.6, -1)
  arc A0 (-16.6, -14) -> (-14.6, -12) centre (-16.6, -12) ccw
  line L18 (-16.6, -14) -> (-63.1, -14)
  arc A1 (-65.1, -12) -> (-63.1, -14) centre (-63.1, -12) ccw
  line L19 (-65.1, -12) -> (-65.1, -1)
  line L20 (-65.1, -1) -> (-64.1, 0)
  line L21 (-64.1, 0) -> (-15.6, 0)
  line L22 (-14.6, -1) -> (-14.6, -12)
  point P0 (-57.1, -4)
  point P1 (-22.6, -4)
  point P2 (-39.85, -4)
  dimension "d215" = 34.5
  dimension "d373" = 4
  constraint horizontal P0 L0.end
  constraint coincident P0 L0.start
  constraint coincident P1 L0.end
  constraint midpoint L1.end L18
  constraint midpoint L1.start L10
  constraint coincident L1 P2
  constraint midpoint L0 P2
  measures "d215" distance of P0 L0.end
  measures "d373" distance of L0 L10
hole "Hole1" at (57.1, -3, 4) at (22.6, -3, 4) direction (0, -1, 0) diameter 6 depth 1 tip angle 180 bodies 5
hole "Hole2" at (22.6, -3, 4) at (57.1, -3, 4) direction (0, 1, 0) diameter 6 depth 1 tip angle 180 bodies 1
ref_plane "WorkPlane1" through (39.85, -8, 7) normal (0, 1, 0) x (0, 0, 1)
sketch "Sketch20" plane through (39.85, -8, 5) normal (0, 1, 0) x (1, 0, 0)
  line L0 (14.25, 1) -> (14.25, -9)
  line L1 (20.25, 1) -> (20.25, -9)
  line L2 (-14.25, 1) -> (-14.25, -9)
  line L3 (-20.25, 1) -> (-20.25, -9)
  arc A0 (-25.25, -7) -> (-23.25, -9) centre (-23.25, -7) ccw
  line L4 (-23.25, -9) -> (23.25, -9)
  arc A1 (23.25, -9) -> (25.25, -7) centre (23.25, -7) ccw
  line L5 (25.25, -7) -> (25.25, 4)
  line L6 (25.25, 4) -> (24.25, 5)
  line L7 (24.25, 5) -> (-24.25, 5)
  line L8 (-24.25, 5) -> (-25.25, 4)
  line L9 (-25.25, 4) -> (-25.25, -7)
  circle A2 centre (17.25, 1) radius 3
  circle A3 centre (-17.25, 1) radius 3
  constraint vertical L2
  constraint vertical L3
  constraint horizontal L0.start L1.start
  constraint horizontal L0.start L2.start
  constraint horizontal L2.start L3.start
  constraint coincident L3.end L4
  constraint coincident L2.end L4
  constraint coincident L0.end L4
  constraint coincident L1.end L4
  constraint vertical L0
  constraint vertical L1
  constraint tangent L0 A2
  constraint coincident L0.start A2
  constraint tangent L1 A2
  constraint tangent L2 A3
  constraint tangent L3 A3
extrude "Extrude24" cut sketch "Sketch20" along normal blind 2 contours L0 L1 L4 A2 | A2 | L2 L3 L4 A3 | A3 bodies 5
sketch "Sketch21" plane through (0, -3, 0) normal (0, -1, 0) x (1, 0, 0)
  line L0 (13.99, 2.25) -> (4.99, 2.25)
  line L1 (4.99, 2.25) -> (4.99, 7.45)
  line L2 (4.99, 7.45) -> (13.99, 7.45)
  line L3 (13.99, 7.45) -> (13.99, 2.25)
  line L4 (65.1, 1) -> (65.54, 1)
  line L5 (65.54, 1) -> (65.54, 17.8)
  line L6 (65.54, 17.8) -> (0.5, 17.8)
  line L7 (0.5, 17.8) -> (0.5, 1)
  line L8 (15.6, 0) -> (64.1, 0)
  line L9 (33.58, 17.8) -> (22.55, 17.8)
  line L10 (21.55, 12.25) -> (34.58, 12.25)
  line L11 (34.58, 12.25) -> (34.58, 8.45)
  line L12 (34.58, 8.45) -> (21.55, 8.45)
  line L13 (21.55, 8.45) -> (21.55, 12.25)
  line L14 (19.32, 3.25) -> (57.82, 3.25)
  line L15 (14.6, 1) -> (15.6, 0)
  line L16 (64.1, 0) -> (65.1, 1)
  line L17 (0.5, 1) -> (14.6, 1)
  circle A0 centre (22.6, 4) radius 3
  circle A1 centre (57.1, 4) radius 3
  dimension "d336" = 5.2
  dimension "d337" = 1
  dimension "d338" = 1
  dimension "d339" = 3.8
  constraint horizontal L10
  constraint vertical L11
  constraint horizontal L12
  constraint vertical L13
  measures "d336" distance of L12 L14
  measures "d337" distance of L9.end L13
  measures "d338" distance of L9.start L11
  measures "d339" distance of L10.end L11.end
extrude "Extrude25" cut sketch "Sketch21" against normal up to surface (3 mm away) contours L10 L11 L12 L13 bodies 1
fillet "Fillet3" radius 1 4 edges at (21.55, -1.5, 8.45) (34.58, -1.5, 8.45) (34.58, -1.5, 12.25) (21.55, -1.5, 12.25) on bodies 1
chamfer "Chamfer11" distance 0.5 angle 45 2 edges at (58.1848, -3, 1.203) (23.6848, -3, 1.203) on bodies 5
chamfer "Chamfer12" distance 0.5 angle 45 8 edges at (28.065, -3, 8.45) (21.8429, -3, 8.7429) (21.55, -3, 10.35) (21.8429, -3, 11.9571) (28.065, -3, 12.25) (34.2871, -3, 11.9571) (34.58, -3, 10.35) (34.2871, -3, 8.7429) on bodies 1
extrude "Extrude32" cut sketch "Sketch4" against normal up to surface (6.45 mm away) from surface at 6.45 contours L1 L44 L45 A8 | L1 L44 L45 L50 bodies 1
extrude "Extrude33" cut sketch "Sketch10" along normal up to surface (2.5 mm away) and the other way blind 1.75 from surface at -2.5 contours L3 L18 L39 L40 | L18 L39 L40 A5 bodies 1
fillet "Fillet6" radius 2 2 edges at (67.54, 14.41, 6.45) (67.54, 18.41, 6.45) on bodies 1
fillet "Fillet6" radius 2.0089 2 edges at (67.54, 16.52, 13.55) (67.54, 20.52, 13.55) on bodies 1
chamfer "Chamfer13" distance 1 angle 45 32 edges at (65.95, 14.41, 0) (61.86, 16.41, 0) (65.95, 18.41, 0) (69.04, 18.41, 2.725) (69.04, 16.41, 6.45) (69.04, 14.41, 2.725) (69.04, 17.1859, 14.05) (69.04, 18.5116, 13.55) (69.04, 19.932, 14.1388) (69.04, 20.52, 16.6795) (68.54, 14.41, 0.5) (68.54, 18.41, 0.5) (67.54, 20.52, 17.8) (64.875, 20.52, 17.8) (61.71, 18.52, 17.8) (66.375, 16.52, 17.8) (36.2005, 12.84, 17.1505) (36.442, 12.1676, 17.392) (37.4776, 11.132, 17.392) (38.15, 10.8905, 17.1505) (39.15, 10.8905, 17.1505) (39.8224, 11.132, 17.392) (40.858, 12.1676, 17.392) (41.0995, 12.84, 17.1505) (41.0995, 13.84, 17.1505) (40.858, 14.5124, 17.392) (39.8224, 15.548, 17.392) (39.15, 15.7895, 17.1505) (38.15, 15.7895, 17.1505) (37.4776, 15.548, 17.392) (36.442, 14.5124, 17.392) (36.2005, 13.84, 17.1505) on bodies 1 4